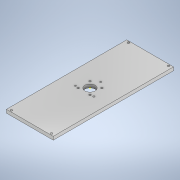
# Autodesk Inventor part: 옆판
Saved by Autodesk Inventor 2020.2 (Build 242310000, 310)
## iProperties
Created: 2020-03-28
Part Number: 옆판
Material: Aluminum 6061-AHC
Document SubType Name: Modeling
Designer: introbot
Density: 2.7 g/cm^3
Appearance: Aluminum - Dark
Mass: 167.073 g
Surface Area: 278.91 cm^2
Volume: 61.8787 cm^3
Author: introbot
Autodesk Inventor part; units mm, degrees
ref_plane "YZ Plane" through (0, 0, 0) normal (1, 0, 0) x (0, 1, 0)
ref_plane "XZ Plane" through (0, 0, 0) normal (0, 1, 0) x (-1, 0, 0)
ref_plane "XY Plane" through (0, 0, 0) normal (0, 0, 1) x (1, 0, 0)
sketch "Sketch1" plane through (0, 0, 0) normal (0, 1, 0) x (-1, 0, 0)
  line L0 (35, 90) -> (-35, 90)
  line L1 (-35, 90) -> (-35, -90)
  line L2 (-35, -90) -> (35, -90)
  line L3 (35, -90) -> (35, 90)
  line L4 (69.6704, 0) -> (-52.4451, 0) projected
  line L5 (0, -129.3465) -> (0, 126.5577) projected
  point P0 (0, 0)
  dimension "d0" = 180
  dimension "d1" = 70
  constraints: 8 end point, 2 parallel, 1 horizontal, 1 perpendicular, 2 other
  measures "d0" distance of L2.end L0.start
  measures "d1" distance of L0.start L0.end
extrude "Extrusion1" add sketch "Sketch1" along normal blind 5
sketch "Sketch2" plane through (0, 5, 0) normal (0, 1, 0) x (1, 0, 0)
  line L0 (-35, 90) -> (-35, -90) projected
  line L1 (35, -90) -> (35, 90) projected
  line L2 (-35, -90) -> (35, -90) projected
  line L3 (-35, -90) -> (35, -90) projected
  line L4 (35, -90) -> (35, 90) projected
  line L5 (35, 90) -> (-35, 90) projected
  line L6 (-35, 90) -> (-35, -90) projected
  line L7 (-49, 0) -> (49, 0) projected
  line L8 (0, 126) -> (0, -126) projected
  point P0 (0, 0)
  point P1 (-30, -87.5)
  point P2 (-30, 87.5)
  point P3 (30, -87.5)
  point P4 (30, 87.5)
  dimension "d4" = 5
  dimension "d5" = 2.5
  constraints: 3 symmetric about line
  measures "d4" distance from line of L0 point (-30, -87.5)
  measures "d5" distance from line of point (-30, -87.5) L2
hole "Hole1" at (-30, 5, -87.5) at (30, 5, 87.5) at (30, 5, -87.5) at (-30, 5, 87.5) direction (0, -1, 0) diameter 3 depth 8.8 tip angle 118
sketch "Sketch3" plane through (0, 5, 0) normal (0, 1, 0) x (1, 0, 0)
  point P0 (0, 0)
hole "Hole2" at (0, 5, 0) direction (0, -1, 0) diameter 15 depth 14.2 tip angle 118
sketch "Sketch4" plane through (0, 5, 0) normal (0, 1, 0) x (1, 0, 0)
  circle A0 centre (0, 0) radius 7.5 projected
  line L0 (35, 90) -> (-35, 90) projected
  line L1 (-35, 90) -> (-35, -90) projected
  line L2 (-35, -90) -> (35, -90) projected
  circle A1 centre (0, 0) radius 12.5
  line L3 (-35, 0) -> (35, 0)
  line L4 (35, -90) -> (35, 90) projected
  line L5 (0, 90) -> (0, -90)
  point P0 (-8.8388, -8.8388)
  point P1 (8.8388, -8.8388)
  point P2 (-8.8388, 8.8388)
  point P3 (8.8388, 8.8388)
  dimension "d42" = 25
  dimension "d45" = 45
  constraints: 4 end point, 4 midpoint, 3 symmetric about line, 1 coincident, 3 other
hole "Hole3" at (-8.8388, 5, 8.8388) at (-8.8388, 5, -8.8388) at (8.8388, 5, -8.8388) at (8.8388, 5, 8.8388) direction (0, -1, 0) diameter 3 end through all
sketch "Sketch5" plane through (0, 5, 0) normal (0, 1, 0) x (1, 0, 0)
  point P0 (0, 0)
sketch "Sketch6" plane through (0, 5, 0) normal (0, 1, 0) x (1, 0, 0)
  point P0 (0, 0)
  point P1 (0, 16)
  point P2 (-13.8564, -8)
  point P3 (0, 0)
  point P4 (13.8564, -8)
  point P5 (0, 0)
  dimension "d30" = 16
  dimension "d33" = 360
  constraints: 2 coincident, 5 other
  measures "d30" distance of point (0, 0) point (0, 16)
hole "Hole4" at (-13.8564, 5, 8) at (13.8564, 5, 8) at (0, 5, -16) direction (0, -1, 0) diameter 2.5 end through all
body "Solid1"
